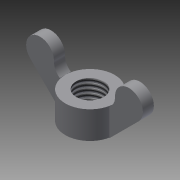
# Autodesk Inventor part: Nut
Saved by Autodesk Inventor 2015 (Build 190159000, 159)
## iProperties
Created: 2018-12-21
Part Number: Nut
Material: Типовые
Document SubType Name: Modeling
Designer: kostya
Density: 1 g/cm^3
Appearance: По умолчанию
Author: kostya
Autodesk Inventor part; units mm, degrees
ref_plane "YZ Plane" through (0, 0, 0) normal (1, 0, 0) x (0, 1, 0)
ref_plane "XZ Plane" through (0, 0, 0) normal (0, 1, 0) x (-1, 0, 0)
ref_plane "XY Plane" through (0, 0, 0) normal (0, 0, 1) x (1, 0, 0)
sketch "Эскиз1" plane through (0, 0, 0) normal (0, 0, 1) x (1, 0, 0)
  circle A0 centre (0, 0) radius 2.5
  circle A1 centre (0, 0) radius 4.5
  dimension "d0" = 5
  dimension "d1" = 9
  constraints: 2 centre point, 2 coincident
  measures "d0" diameter of A0
  measures "d1" diameter of A1
extrude "Выдавливание1" add sketch "Эскиз1" along normal blind 5
sketch "Эскиз2" plane through (0, 0, 0) normal (0, 1, 0) x (-1, 0, 0)
  line L0 (4.5, 0) -> (4.5, 5) projected
  line L1 (4.5, 5) -> (-4.5, 5) projected
  line L2 (4.5, 0) -> (9.8918, 5.3918)
  line L3 (4.5, 0) -> (14.667, 0) construction
  arc A0 (9.8918, 5.3918) -> (5.5593, 7.0075) centre (8.0946, 7.1891) ccw
  arc A1 (4.5, 5) -> (5.5528, 7.1891) centre (3.1205, 7.0112) ccw
  line L4 (0, 5) -> (0, 0) construction
  line L5 (-4.5, 0) -> (-4.5, 5)
  line L6 (-4.5, 0) -> (-9.8918, 5.3918)
  arc A2 (-5.5593, 7.0075) -> (-9.8918, 5.3918) centre (-8.0946, 7.1891) ccw
  arc A3 (-5.5528, 7.1891) -> (-4.5, 5) centre (-3.1205, 7.0112) ccw
  point P0 (6.2973, 8.9864)
  dimension "d4" = 45
  constraints: 13 point on circle, 10 end point, 6 symmetric about line, 4 centre point, 1 coincident, 1 horizontal, 1 midpoint, 1 tangent, 1 vertical, 2 other
  measures "d4" angle of L3 L2
extrude "Выдавливание2" add sketch "Эскиз2" along normal mid plane 2 contours L5 L6 A2 A3 | L0 A1 A0 L2
thread "Резьба1" size "M5x0.8" class "6H" standard "ANSI Metric M Profile" full length
